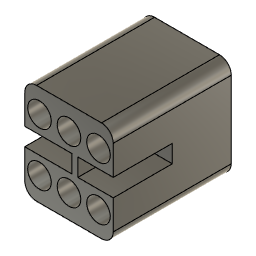
PartnerPDM Connector Rev1 (Autodesk Fusion 360 design; units mm, degrees)
Autodesk Fusion 360 part; units mm, degrees
sketch "Sketch1" plane through (0, 0, 0) normal (0, 1, 0) x (1, 0, 0)
  line L0 (0.7695, -2.3211) -> (15.7695, -2.3211)
  line L1 (15.7695, -2.3211) -> (15.7695, 4.6789)
  line L2 (0.7695, 4.6789) -> (0.7695, -2.3211)
  line L3 (15.7695, 7.6789) -> (15.7695, 14.6789)
  line L4 (0.7695, 14.6789) -> (0.7695, 7.6789)
  line L5 (15.7695, 14.6789) -> (0.7695, 14.6789)
  line L6 (9.7695, 4.6789) -> (9.7695, 7.6789)
  line L7 (8.7695, 7.6789) -> (8.7695, 4.6789)
  circle A0 centre (8.2695, 1.6789) radius 2
  line L8 (15.7695, 4.6789) -> (9.7695, 4.6789)
  line L9 (8.7695, 4.6789) -> (0.7695, 4.6789)
  line L10 (0.7695, 7.6789) -> (8.7695, 7.6789)
  line L11 (9.7695, 7.6789) -> (15.7695, 7.6789)
  circle A1 centre (13.2695, 1.6789) radius 2
  circle A2 centre (3.2695, 1.6789) radius 2
  circle A3 centre (8.2695, 10.6789) radius 2
  circle A4 centre (13.2695, 10.6789) radius 2
  circle A5 centre (3.2695, 10.6789) radius 2
  circle A6 centre (-6.7305, 1.6789) radius 1
  circle A7 centre (-11.7305, 1.6789) radius 1
  circle A8 centre (-16.7305, 1.6789) radius 1
  line L12 (-4.7305, -1.3211) -> (-18.7305, -1.3211)
  line L13 (-18.7305, -1.3211) -> (-18.7305, 3.6789)
  line L14 (-18.7305, 3.6789) -> (-4.7305, 3.6789)
  line L15 (-4.7305, 3.6789) -> (-4.7305, -1.3211)
  circle A9 centre (-6.7305, 10.6789) radius 1
  circle A10 centre (-16.7305, 10.6789) radius 1
  circle A11 centre (-11.7305, 10.6789) radius 1
  line L16 (-4.7305, 8.6789) -> (-18.7305, 8.6789)
  line L17 (-4.7305, 13.6789) -> (-4.7305, 8.6789)
  line L18 (-18.7305, 13.6789) -> (-4.7305, 13.6789)
  line L19 (-18.7305, 8.6789) -> (-18.7305, 13.6789)
  line L20 (20.7695, 3.6789) -> (35.7695, 3.6789)
  line L21 (35.7695, 3.6789) -> (35.7695, 8.6789)
  line L22 (35.7695, 8.6789) -> (20.7695, 8.6789)
  line L23 (20.7695, 8.6789) -> (20.7695, 3.6789)
  dimension "d1" = 15
  dimension "d2" = 7
  dimension "d3" = 15
  dimension "d4" = 7
  dimension "d6" = 6
  dimension "d7" = 4
  dimension "d8" = 4
  dimension "d9" = 4
  dimension "d10" = 5
  dimension "d11" = 5
  dimension "d12" = 4
  dimension "d13" = 2.5
  dimension "d14" = 4
  dimension "d15" = 4
  dimension "d16" = 4
  dimension "d17" = 5
  dimension "d18" = 5
  dimension "d21" = 2
  dimension "d22" = 2
  dimension "d23" = 2
  dimension "d24" = 14
  dimension "d25" = 5
  dimension "d27" = 1
  dimension "d29" = 5
  dimension "d30" = 5
  dimension "d31" = 3
  dimension "d32" = 20.5
  dimension "d33" = 2
  dimension "d34" = 2
  dimension "d35" = 2
  dimension "d36" = 2
  dimension "d37" = 14
  dimension "d38" = 5
  dimension "d39" = 5
  dimension "d40" = 5
  dimension "d41" = 2
  dimension "d42" = 2
  dimension "d43" = 1
  dimension "d49" = 5
  dimension "d50" = 15
  dimension "d51" = 20
  constraint horizontal L0
  constraint vertical L1
  constraint horizontal L8
  constraint vertical L2
  constraint horizontal L10
  constraint vertical L3
  constraint horizontal L5
  constraint vertical L4
  constraint vertical L6
  constraint vertical L7
  constraint coincident L7.end L8
  constraint collinear L8 L9
  constraint coincident L6.end L10
  constraint collinear L10 L11
  constraint horizontal L12
  constraint vertical L13
  constraint horizontal L14
  constraint vertical L15
  constraint horizontal L16
  constraint vertical L19
  constraint horizontal L18
  constraint vertical L17
  constraint horizontal L20
  constraint vertical L21
  constraint horizontal L22
  constraint vertical L23
  measures "d1" distance of L0.start L0.end
  measures "d2" distance of L0.start L2.start
  measures "d3" distance of L4.end L3.start
  measures "d4" distance of L4.start L4.end
  measures "d6" distance of L1.end L6
  measures "d7" diameter of A0
  measures "d8" diameter of A1
  measures "d9" diameter of A2
  measures "d10" distance of A0.centre A1.centre
  measures "d11" distance of A0.centre A2.centre
  measures "d12" distance of L0 A2.centre
  measures "d13" distance of L2 A2.centre
  measures "d14" diameter of A3
  measures "d15" diameter of A4
  measures "d16" diameter of A5
  measures "d17" distance of A3.centre A4.centre
  measures "d18" distance of A5.centre A3.centre
  measures "d21" diameter of A6
  measures "d22" diameter of A7
  measures "d23" diameter of A8
  measures "d24" distance of L12.start L12.end
  measures "d25" distance of L12.end L13.end
  measures "d27" vertical distance of L2.start L14.end
  measures "d29" distance of A7.centre A8.centre
  measures "d30" distance of A6.centre A7.centre
  measures "d31" distance of A8.centre L12
  measures "d32" horizontal distance of L0.end L12.start
  measures "d33" distance of A8.centre L13
  measures "d34" diameter of A9
  measures "d35" diameter of A11
  measures "d36" diameter of A10
  measures "d37" distance of L16.start L16.end
  measures "d38" distance of L16.end L18.start
  measures "d39" distance of A10.centre A11.centre
  measures "d40" distance of A9.centre A11.centre
  measures "d41" distance of A10.centre L16
  measures "d42" distance of A10.centre L19
  measures "d43" distance of L5 L17.start
  measures "d49" distance of L20.end L21.end
  measures "d50" distance of L20.start L20.end
  measures "d51" horizontal distance of L1.end L20.end
extrude "Extrude4" add sketch "Sketch1" along normal blind 20 contours L0 L1 L2 L3 L4 L5 L6 L7 L8 L9 L10 L11 makes body 1
extrude "Extrude5" add sketch "Sketch1" along normal blind 1.8 separate body contours L12 L13 L14 L15 | L16 L17 L18 L19 makes body 2 at (-11.7056, 0, 0.6535) makes body 3 at (-11.7555, 0, -13.0113)
move_body "Move2" bodies 2 3 to x (1, 0, 0) y (0, 1, 0) z (0, 0, 1) at (20, 6, 0)
extrude "Extrude6" add sketch "Sketch1" along normal blind 10 separate body contours L20 L21 L22 L23 makes body 4
move_body "Move4" bodies 4 to x (1, 0, 0) y (0, 1, 0) z (0, 0, 1) at (0, 10, 0)
move_body "Move5" bodies 4 to x (1, 0, 0) y (0, 1, 0) z (0, 0, 1) at (-20, 0, 0)
combine "Combine1" operation add target body 1 tool bodies 3 4 2
fillet "Fillet5" radius 2 1 edges at (15.7695, 10, -14.6789) on bodies 1
fillet "Fillet6" radius 2 1 edges at (0.7695, 10, -14.6789) on bodies 1
fillet "Fillet7" radius 2 1 edges at (0.7695, 10, 2.3211) on bodies 1
fillet "Fillet8" radius 2 1 edges at (15.7695, 10, 2.3211) on bodies 1
